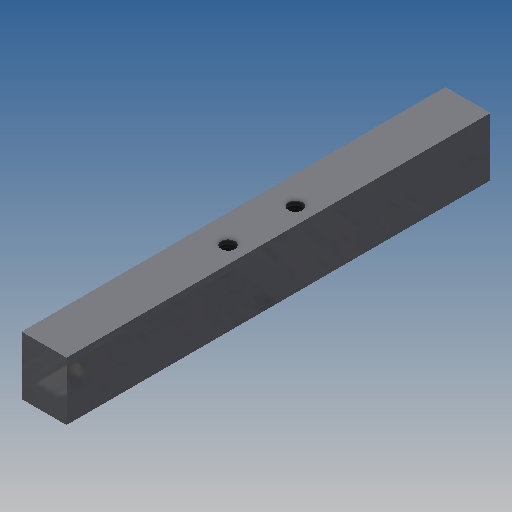
# Autodesk Inventor part: PWTR-0041
Saved by Autodesk Inventor 2021.1 (Build 251245000, 245)
## iProperties
Shininess: 64.0
Length Units: 11269
Angle Units: 11279
Time Units: 11290
Mass Units: 11284
Length Display Precision: 3
Angle Display Precision: 2
Compacted: True
Part Number: PWTR-0041
Document SubType Name: Modeling
Created: 2003-02-04
Designer: B. BOGAN
Material: Stainless Steel, 303
Description: Trowel Support
Density: 7.75 g/cm^3
Appearance: Metal-Steel (Polished)
Mass: 183.226 g
Surface Area: 82.7529 cm^2
Volume: 23.642 cm^3
Vendor: Design Specific
Density: 0.0
Volumn: 0.0
Area: 0.0
PropertySet Name: Model Information
Control State: 0
Master: False
Checked Out: False
Title: TROWEL SUPPORT
Author: B. BOGAN
Revision Number: B
Autodesk Inventor part; units mm, degrees
ref_plane "YZ Plane" through (0, 0, 0) normal (1, 0, 0) x (0, 1, 0)
ref_plane "XZ Plane" through (0, 0, 0) normal (0, 1, 0) x (-1, 0, 0)
ref_plane "XY Plane" through (0, 0, 0) normal (0, 0, 1) x (1, 0, 0)
sketch "Sketch1" plane through (0, 0, 0) normal (0, 0, 1) x (1, 0, 0)
  line L0 (-8.5, 0) -> (8.5, 0)
  line L1 (8.5, 0) -> (8.5, 22)
  line L2 (8.5, 22) -> (-8.5, 22)
  line L3 (-8.5, 22) -> (-8.5, 0)
  point P0 (0, 0)
  point P1 (0, 0)
  dimension "d0" = 22
  dimension "d1" = 17
  constraints: 8 end point, 2 parallel, 1 coincident, 1 horizontal, 1 midpoint, 1 perpendicular
  measures "d0" distance between parallel lines of L2 L0
  measures "d1" distance between parallel lines of L1 L3
extrude "Extrusion1" add sketch "Sketch1" along normal mid plane 160
sketch "Sketch2" plane through (-8.5, 22, -80) normal (0, 1, 0) x (1, 0, 0)
  line L0 (17, 0) -> (17, -160) projected
  line L1 (10.65, -92.7) -> (10.65, -80)
  point P0 (17, -80)
  dimension "d4" = 6.35
  dimension "d16" = 12.7
  constraints: 2 end point, 1 horizontal alignment, 1 midpoint, 1 vertical
  measures "d4" distance from line of L1.start L0
  measures "d16" distance of L1.start L1.end
hole "Hole1" at (2.15, 22, 12.7) direction (0, -1, 0) diameter 5.2578 end through all thread size "1/4-20 UNC" class "2B" standard "ANSI Unified Screw Threads"
pattern_linear "Rectangular Pattern1" count 2 spacing 25.4 along (0, 0, -1) of "Hole1"
body "Solid1"
